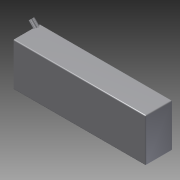
# Autodesk Inventor part: LiPoBattery
Saved by Autodesk Inventor 2011 SP2 (Build 150309200, 309)
## iProperties
Created: 2015-10-13
Part Number: LiPoBattery
Document SubType Name: Modeling
Designer: Ernest
Density: 1 g/cm^3
Author: Ernest
Autodesk Inventor part; units mm, degrees
ref_plane "YZ Plane" through (0, 0, 0) normal (1, 0, 0) x (0, 1, 0)
ref_plane "XZ Plane" through (0, 0, 0) normal (0, 1, 0) x (-1, 0, 0)
ref_plane "XY Plane" through (0, 0, 0) normal (0, 0, 1) x (1, 0, 0)
sketch "Sketch1" plane through (0, 0, 0) normal (0, 0, 1) x (1, 0, 0)
  line L0 (0, 0) -> (138, 0)
  line L1 (138, 0) -> (138, 28)
  line L2 (138, 28) -> (0, 28)
  line L3 (0, 28) -> (0, 0)
  dimension "d0" = 138
  dimension "d1" = 28
  constraints: 8 end point, 2 parallel, 1 horizontal, 1 perpendicular
  measures "d0" distance of L0.start L0.end
  measures "d1" distance of L2.end L0.start
extrude "Extrusion1" add sketch "Sketch1" along normal blind 45
ref_plane "Work Plane1" through (0, 28, 45) normal (0.7071068, 0, -0.7071068) x (0, 1, 0)
sketch "Sketch2" plane through (0, 28, 45) normal (0.7071068, 0, -0.7071068) x (0, 1, 0)
  line L0 (-28, 0) -> (0, 0) projected
  circle A0 centre (-3.049, 0) radius 1.5
  circle A1 centre (-5.7153, 0) radius 1.5
  circle A2 centre (-7.2153, 0.7211) radius 0.5
  circle A3 centre (-4.3663, 1.3485) radius 0.5
  circle A4 centre (-4.3663, -1.3706) radius 0.5
  point P0 (-28, -31.8198)
  dimension "d5" = 3
  dimension "d6" = 3
  dimension "d7" = 1
  dimension "d8" = 1
  dimension "d9" = 1
  constraints: 5 centre point, 2 point on line
  measures "d5" diameter of A0
  measures "d6" diameter of A1
  measures "d7" diameter of A2
  measures "d8" diameter of A3
  measures "d9" diameter of A4
extrude "Extrusion2" add sketch "Sketch2" along normal mid plane 12.5 contours A1 A0 A3 L0 | A1 A0 L0 | L0 A0 A1 | L0 A0 A4 A1 | A0 A1 A4 L0 | L0 A1 A2 A3 A0 | A3 A0 | A0 A3 A1 | A4 A1 A0 | A0 A4 | A3 A1 | A1 A4 | A2 A1 | A1 A2 picked at (-4.3907, 1.3671) picked at (-4.3952, -1.3761)
fillet "Fillet1" radius 1 13 edges at (0, 10.3924, 45) (69, 28, 45) (69, 0, 45) (0, 27.2255, 45) (0, 28, 22.5) (0, 0, 22.5) (0, 14, 0) (69, 28, 0) (138, 28, 22.5) (138, 14, 45) (138, 0, 22.5) (138, 14, 0) (69, 0, 0)
body "Solid1"
